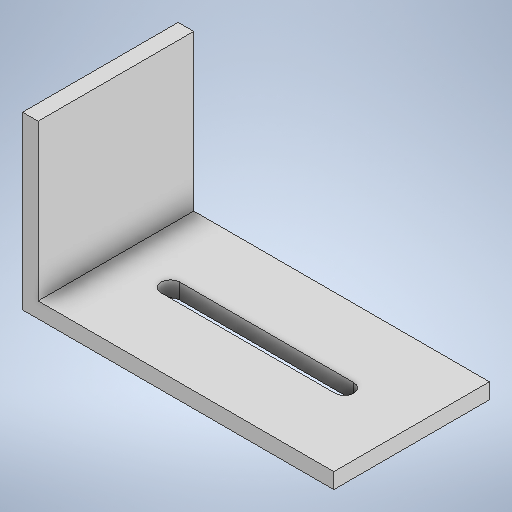
# Autodesk Inventor part: Horonyrogzito_b
Saved by Autodesk Inventor 2025.2 (Build 292293000, 293)
## iProperties
Created: 2025-08-22
Part Number: Horonyrogzito_b
Material: Generic
Document SubType Name: Modeling
Designer: MB
Density: 1 g/cm^3
Appearance: Default
Author: MB
Autodesk Inventor part; units mm, degrees
ref_plane "YZ Plane" through (0, 0, 0) normal (1, 0, 0) x (0, 1, 0)
ref_plane "XZ Plane" through (0, 0, 0) normal (0, 1, 0) x (-1, 0, 0)
ref_plane "XY Plane" through (0, 0, 0) normal (0, 0, 1) x (1, 0, 0)
sketch "Sketch1" plane through (0, 0, 0) normal (0, 1, 0) x (-1, 0, 0)
  line L0 (0, 0) -> (-100, 0)
  line L1 (-100, 0) -> (-100, 50)
  line L2 (-100, 50) -> (0, 50)
  line L3 (0, 50) -> (0, 0)
  dimension "d0" = 100
  dimension "d1" = 50
  constraints: 8 end point, 2 parallel, 1 horizontal, 1 perpendicular
  measures "d0" distance of L1.end L2.end
  measures "d1" distance of L0.end L1.end
extrude "Extrusion1" add sketch "Sketch1" along normal blind 5
sketch "Sketch3" plane through (0, 5, 0) normal (0, 1, 0) x (1, 0, 0)
  line L0 (0, -50) -> (100, -50) projected
  line L1 (0, 0) -> (5, 0)
  line L2 (5, 0) -> (5, -50)
  line L3 (5, -50) -> (0, -50)
  line L4 (0, -50) -> (0, 0)
  dimension "d14" = 5
  constraints: 8 end point, 2 parallel, 1 horizontal, 1 perpendicular, 1 point on line
  measures "d14" distance of L2.end L3.end
extrude "Extrusion2" add sketch "Sketch3" along normal blind 50
sketch "Sketch4" plane through (0, 5, 0) normal (0, 1, 0) x (1, 0, 0)
  line L0 (5, 0) -> (5, -50) projected
  line L1 (5, -50) -> (100, -50) construction
  line L2 (100, -50) -> (100, 0) construction
  line L3 (100, 0) -> (5, 0) construction
  arc A0 (78.411, -28) -> (78.411, -22) centre (78.411, -25) ccw
  arc A1 (22.5222, -22) -> (22.5222, -28) centre (22.5222, -25) ccw
  line L4 (22.5222, -22) -> (78.411, -22)
  line L5 (78.411, -28) -> (22.5222, -28)
  point P0 (0, 0)
  point P1 (100, -25)
  dimension "d30" = 6
  dimension "d31" = 6
  dimension "d32" = 25
  constraints: 4 end point, 4 point on circle, 2 centre point, 1 horizontal, 1 midpoint, 1 tangent
  measures "d30" diameter of A0
  measures "d31" diameter of A1
  measures "d32" distance from line of L1 A0.centre
extrude "Extrusion3" cut sketch "Sketch4" against normal up to surface (5 mm away)
body "Solid1"
